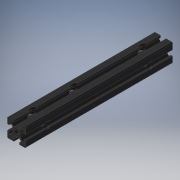
# Autodesk Inventor part: HFS5-2020-160-AH24-BH136-Z6-XA20-XB65-XC140
Saved by Autodesk Inventor 2019 (Build 230136000, 136)
## iProperties
Created: 2024-09-09
Part Number: HFS5-2020-160-AH24-BH136-Z6-XA20-XB65-XC140
Material: Generic
Catalog Web Link: www.cadenas.de
Description: NFS5-2020, NFSB5-2020, HFS5-2020, HFSB5-2020, CAF5-2020, HFSY5-2020, NFSF5-2020, HFSF5-2020, HFSFB5-2020, NFST5-2020, HFST5-2020, HFSTB5-2020, HFSH5-2020, HFSC5-2020-HFS5 Series Aluminum Extrusions 20 Square -1 Slot-
Vendor: MISUMI
Document SubType Name: Modeling
Designer: psAdmin
Manufacturer: MISUMI
Mass: 27.8589 g
Surface Area: 278.381 cm^2
Volume: 27.8589 cm^3
Density: 1 g/cm^3
Appearance: PSOLRGB-175-175-175
Category: PARTsolutions
Company: MISUMI
Title: HFS5-2020-160-AH24-BH136-Z6-XA20-XB65-XC140
Author: Cadenas PARTsolutions
Comments: HFS5 Series Aluminum Extrusions 20 Square -1 Slot-
PSOL_IDENT_0: {$CADENAS_DATA/23d-libs/misumi/metric/38_al_extrusions_blackets/5/hfs5_2020.prj},737 {VTYP=3D},{NB=H
PSOL_IDENT_1: FS5-2020-160-AH24-BH136-Z6-XA20-XB65-XC140},{LINA=HFS5-2020-160-AH24-BH136-Z6-XA20-XB65-XC140},{NN=N
PSOL_IDENT_2: FS5-2020, NFSB5-2020, HFS5-2020, HFSB5-2020, CAF5-2020, HFSY5-2020, NFSF5-2020, HFSF5-2020, HFSFB5-2
PSOL_IDENT_3: 020, NFST5-2020, HFST5-2020, HFSTB5-2020, HFSH5-2020, HFSC5-2020},{DATE=08.05.2023 08:39:06},{GEOMDA
PSOL_IDENT_4: TE=27.07.2021 03:20:00},{VERSION=},{LINEID=150},{WBVAR=L,ALT1,ALT2,ALT4,ALT5,CP5,DL5,DR5,ALT6,ALT9,A
PSOL_IDENT_5: LT10,ALT11,HP6,NHL6,DL6,NHR6,DR6,ALT7,ALT8,NH9,AH,BH,CH,DH,EH,NH10,AV,BV,CV,DV,EV,NH11,AP,BP,CP,DP,E
PSOL_IDENT_6: P,ALT12,ALT13,Z,NH12,XA,XB,XC,XD,XE,NH13,YA,YB,YC,YD,YE,ALT16,HP16,DL16,DR16,ALT17,HQ17,JLP,ALT20},{
PSOL_IDENT_7: WBNUMERIC=L,NH9,AH,BH,CH,DH,EH,NH10,AV,BV,CV,DV,EV,NH11,AP,BP,CP,DP,EP,NH12,XA,XB,XC,XD,XE,NH13,YA,Y
PSOL_IDENT_8: B,YC,YD,YE,HQ17,JLP}  {NB=HFS5-2020-160-AH24-BH136-Z6-XA20-XB65-XC140},{LINA=HFS5-2020-160-AH24-BH13
PSOL_IDENT_9: 6-Z6-XA20-XB65-XC140},{KT=DUMMY},{PN=HFS5-2020-160-AH24-BH136-Z6-XA20-XB65-XC140},{TPS=HFS5-2020},{M
PSOL_IDENT_10: AT=A6N01SS-T5 Aluminum Alloy or 6005A-T5 Aluminum Alloy},{ST=Clear Anodize},{FRMW=20},{FRMH=20},{FRD=
PSOL_IDENT_11: 4.2},{L=160},{MASS=0.5},{SA=183},{LX=0.742x10^4},{LY=0.742x10^4},{ALT1=},{M1=0},{DPL1=0},{DPR1=0},{A
PSOL_IDENT_12: LT1PN=},{ALT2=},{ALT2ALG= '','w/o End Tapping (Heli-Coil Insert)','LHP','with LHP (Tapping on the Le
PSOL_IDENT_13: ft (Heli-Coil Insert))','RHP','with RHP (Tapping on the Right (Heli-Coil Insert))','HPW','with HPW (
PSOL_IDENT_14: Tapping on Both Ends (Heli-Coil Insert))' },{M2=0},{DP2=0},{ALT2PN=},{ALT4=},{ALT4ALG= '', 'w/o SC (
PSOL_IDENT_15: High Precision Cut)', 'SC', 'with SC (High Precision Cut)' },{ALT4PN=},{ALT5=},{ALT5ALG= '','w/o 45
PSOL_IDENT_16: Degree Cut','1','with 45 Degree Cut' },{CP5=},{CP5ALG= '','N/A' },{DL5=},{DL5ALG= '','N/A' },{DR5=},
PSOL_IDENT_17: {DR5ALG= '','N/A' },{FRMLALT5=0},{FRMRALT5=0},{ALT5PN=},{ALT6=},{ALT6ALG= '','w/o Fastening Location
PSOL_IDENT_18: Wrench Access Hole Alterations','1','with Fastening Location Wrench Access Hole Alterations' },{ALT
PSOL_IDENT_19: 9=1},{ALT9ALG= '','w/o Location Specified Wrench Access Hole Alteratons (Horizontal)','1','with Loca
PSOL_IDENT_20: tion Specified Wrench Access Hole Alteratons (Horizontal)' },{ALT10=},{ALT10ALG= '','w/o Location Sp
PSOL_IDENT_21: ecified Wrench Access Hole Alteratons (Vertical)','1','with Location Specified Wrench Access Hole Al
PSOL_IDENT_22: teratons (Vertical)' },{ALT11=},{ALT11ALG= '','w/o Location Specified Wrench Access Hole Alteratons
PSOL_IDENT_23: (Crisscross)','1','with Location Specified Wrench Access Hole Alteratons (Crisscross)' },{HP6=},{HP6
PSOL_IDENT_24: ALG= '','N/A' },{NHL6=},{NHL6ALG= '','N/A' },{DL6=},{DL6ALG= '','N/A' },{NHR6=},{NHR6ALG= '','N/A' }
PSOL_IDENT_25: ,{DR6=},{DR6ALG= '','N/A' },{HL6=0.000},{HL6D=0},{HR6=0.000},{HR6D=0},{J6=0},{J6D=0},{K6=0},{K6D=0},
PSOL_IDENT_26: {DD6=7.35},{DD6ALG=7.35},{ALT7=},{ALT7ALG= '','N/A' },{ALT8=},{ALT8ALG= '','N/A' },{ALT678PN=},{NH9=
PSOL_IDENT_27: 2},{NH9MAX=5},{NH9ALG=[1:5/1]},{AH=24.0},{AHMIN=7},{AHMAX=143.5},{AHALG=[7:143.5/0.5]},{BH=136.0},{B
PSOL_IDENT_28: HMIN=33.5},{BHMAX=153},{BHALG=[33.5:153/0.5]},{CH=0.0},{CHMIN=145.5},{CHMAX=162.5},{CHALG=[0]},{DH=0
PSOL_IDENT_29: .0},{DHMIN=9.5},{DHMAX=172},{DHALG=[0]},{EH=0.0},{EHMIN=9.5},{EHMAX=153},{EHALG=[0]},{NH10=0},{NH10M
PSOL_IDENT_30: AX=5},{NH10ALG=[0]},{AV=0.0},{AVMIN=7},{AVMAX=162.5},{AVALG=[0]},{BV=0.0},{BVMIN=9.5},{BVMAX=172},{B
PSOL_IDENT_31: VALG=[0]},{CV=0.0},{CVMIN=9.5},{CVMAX=181.5},{CVALG=[0]},{DV=0.0},{DVMIN=9.5},{DVMAX=191},{DVALG=[0]
PSOL_IDENT_32: },{EV=0.0},{EVMIN=9.5},{EVMAX=153},{EVALG=[0]},{NH11=0},{NH11MAX=5},{NH11ALG=[0]},{AP=0.0},{APMIN=7}
PSOL_IDENT_33: ,{APMAX=162.5},{APALG=[0]},{BP=0.0},{BPMIN=9.5},{BPMAX=172},{BPALG=[0]},{CP=0.0},{CPMIN=9.5},{CPMAX=
PSOL_IDENT_34: 181.5},{CPALG=[0]},{DP=0.0},{DPMIN=9.5},{DPMAX=191},{DPALG=[0]},{EP=0.0},{EPMIN=9.5},{EPMAX=153},{EP
PSOL_IDENT_35: ALG=[0]},{ALT9PN=-AH24-BH136},{ALT10PN=},{ALT11PN=},{ALT91011PN=-AH24-BH136},{ALT12=1},{ALT12ALG= ''
PSOL_IDENT_36: ,'w/o Counterbore Hole in Specified Position (Vertical)','1','with Counterbore Hole in Specified Pos
PSOL_IDENT_37: ition (Vertical)' },{ALT13=},{ALT13ALG= '','w/o Counterbore Hole in Specified Position (Horizontal)'
PSOL_IDENT_38: ,'1','with Counterbore Hole in Specified Position (Horizontal)' },{Z=6},{ZALG='5','5','6','6'},{DD12=
PSOL_IDENT_39: 6.5},{DD112=11.0},{NH12=3},{NH12MAX=5},{NH12ALG=[1:5/1]},{XA=20.0},{XAMIN=7},{XAMAX=127},{XAALG=[7:1
PSOL_IDENT_40: 27/0.5]},{XB=65.0},{XBMIN=33},{XBMAX=140},{XBALG=[33:140/0.5]},{XC=140.0},{XCMIN=78},{XCMAX=153},{XC
PSOL_IDENT_41: ALG=[78:153/0.5]},{XD=0.0},{XDMIN=153},{XDMAX=166},{XDALG=[0]},{XE=0.0},{XEMIN=13},{XEMAX=153},{XEAL
PSOL_IDENT_42: G=[0]},{NH13=0},{NH13MAX=5},{NH13ALG=[0]},{YA=0.0},{YAMIN=7},{YAMAX=166},{YAALG=[0]},{YB=0.0},{YBMIN=
PSOL_IDENT_43: 13},{YBMAX=179},{YBALG=[0]},{YC=0.0},{YCMIN=13},{YCMAX=192},{YCALG=[0]},{YD=0.0},{YDMIN=13},{YDMAX=2
PSOL_IDENT_44: 05},{YDALG=[0]},{YE=0.0},{YEMIN=13},{YEMAX=153},{YEALG=[0]},{ALT12PN=-XA20-XB65-XC140},{ALT13PN=},{A
PSOL_IDENT_45: LT1213PN=-Z6-XA20-XB65-XC140},{ALT16=},{ALT16ALG= '','w/o M Type Hole Alteration','1','with M Type H
PSOL_IDENT_46: ole Alteration' },{HP16=},{HP16ALG= '','N/A' },{DL16=},{DL16ALG= '','N/A' },{DR16=},{DR16ALG= '','N/
PSOL_IDENT_47: A' },{H116=0},{D16=0.0},{ALT16PN=},{ALT17=},{ALT17ALG= '','w/o L Type Hole Alteration (Top)','1','wi
PSOL_IDENT_48: th L Type Hole Alteration (Top)' },{HQ17=0},{HQ17ALG=0},{JLP=0},{JLPMIN=4.9},{JLPMAX=0},{JLPALG=[0]}
PSOL_IDENT_49: ,{L17=0},{D17=0.0},{ALT17PN=},{ALT20=},{ALT20PN=},{ERRORALT01=OK},{ERRORALT02=OK},{ERRORALT05=OK},{E
PSOL_IDENT_50: RRORALT06091=OK},{ERRORALT06092=OK},{ERRORALT06093=OK},{ERRORALT06094=OK},{ERRORALT06101=OK},{ERRORA
PSOL_IDENT_51: LT06102=OK},{ERRORALT06103=OK},{ERRORALT06104=OK},{ERRORALT06111=OK},{ERRORALT06112=OK},{ERRORALT061
PSOL_IDENT_52: 13=OK},{ERRORALT06114=OK},{ERRORALT06121=OK},{ERRORALT06122=OK},{ERRORALT06123=OK},{ERRORALT06124=OK
PSOL_IDENT_53: },{ERRORALT06131=OK},{ERRORALT06132=OK},{ERRORALT06133=OK},{ERRORALT06134=OK},{ERRORALT0616=OK},{ERR
PSOL_IDENT_54: ORALT06171=OK},{ERRORALT06172=OK},{ERRORALT06173=OK},{ERRORALT0911=OK},{ERRORALT0913=OK},{ERRORALT09
PSOL_IDENT_55: 16=OK},{ERRORALT0917=OK},{ERRORALT1011=OK},{ERRORALT1012=OK},{ERRORALT1016=OK},{ERRORALT1017=OK},{ER
PSOL_IDENT_56: RORALT1112=OK},{ERRORALT1113=OK},{ERRORALT1116=OK},{ERRORALT1117=OK},{ERRORALT1216=OK},{ERRORALT1217=
PSOL_IDENT_57: OK},{ERRORALT1316=OK},{ERRORALT1317=OK},{ERRORALT1617=OK},{ERRORPN=},{TFW=0}
NB: HFS5-2020-160-AH24-BH136-Z6-XA20-XB65-XC140
NN: NFS5-2020, NFSB5-2020, HFS5-2020, HFSB5-2020, CAF5-2020, HFSY5-2020, NFSF5-2020, HFSF5-2020, HFSFB5-2020, NFST5-2020, HFST5-2020, HFSTB5-2020, HFSH5-2020, HFSC5-2020
NT: HFS5 Series Aluminum Extrusions 20 Square -1 Slot-
NBSYN: $PN.
LINA: HFS5-2020-160-AH24-BH136-Z6-XA20-XB65-XC140
CATALOG: Misumi
PN: HFS5-2020-160-AH24-BH136-Z6-XA20-XB65-XC140
TPS: HFS5-2020
MAT: A6N01SS-T5 Aluminum Alloy or 6005A-T5 Aluminum Alloy
ST: Clear Anodize
L: 160
MASS: 0.5
SA: 183
LX: 0.742x10^4
LY: 0.742x10^4
ALT1: w/o End Tapping
M1: 0
DPL1: 0
DPR1: 0
ALT2: w/o End Tapping (Heli-Coil Insert)
M2: 0
DP2: 0
ALT4: w/o SC (High Precision Cut)
ALT5: w/o 45 Degree Cut
CP5: N/A
DL5: N/A
DR5: N/A
ALT6: w/o Fastening Location Wrench Access Hole Alterations
ALT9: with Location Specified Wrench Access Hole Alteratons (Horizontal)
ALT10: w/o Location Specified Wrench Access Hole Alteratons (Vertical)
ALT11: w/o Location Specified Wrench Access Hole Alteratons (Crisscross)
HP6: N/A
NHL6: N/A
DL6: N/A
NHR6: N/A
DR6: N/A
HL6D: 0
HR6D: 0
J6D: 0
K6D: 0
DD6: 7.35
ALT7: N/A
ALT8: N/A
NH9: 2
AH: 24
BH: 136
CH: 0
DH: 0
EH: 0
NH10: 0
AV: 0
BV: 0
CV: 0
DV: 0
EV: 0
NH11: 0
AP: 0
BP: 0
CP: 0
DP: 0
EP: 0
ALT12: with Counterbore Hole in Specified Position (Vertical)
ALT13: w/o Counterbore Hole in Specified Position (Horizontal)
Z: 6
DD12: 6.5
DD112: 11
NH12: 3
XA: 20
XB: 65
XC: 140
XD: 0
XE: 0
NH13: 0
YA: 0
YB: 0
YC: 0
YD: 0
YE: 0
ALT16: w/o M Type Hole Alteration
HP16: N/A
DL16: N/A
DR16: N/A
H116: 0
D16: 0
ALT17: w/o L Type Hole Alteration (Top)
HQ17: 0
JLP: 0
D17: 0
ALT20: w/o CW (End Face C Chamfering)
SUPPLIER: MISUMI
ARTICLENO: HFS5-2020-160-AH24-BH136-Z6-XA20-XB65-XC140
BOMINFO: HFS5-2020-160-AH24-BH136-Z6-XA20-XB65-XC140
CREATOR: CADENAS GmbH
Autodesk Inventor part; units mm, degrees
sketch "Sketch_1" plane through (0, 0, 0) normal (0, 0, 1) x (1, 0, 0)
  line L0 (-10, -3) -> (-10, -9)
  arc A0 (-10, -9) -> (-9, -10) centre (-9, -9) ccw
  line L1 (-9, -10) -> (-3, -10)
  line L2 (-3, -10) -> (-3, -8)
  line L3 (-3, -8) -> (-6, -8)
  line L4 (-6, -8) -> (-6, -7.0607)
  line L5 (-6, -7.0607) -> (-2.9393, -4)
  line L6 (-2.9393, -4) -> (-0.5196, -4)
  line L7 (-0.5196, -4) -> (0, -3.7)
  line L8 (0, -3.7) -> (0.5196, -4)
  line L9 (0.5196, -4) -> (2.9393, -4)
  line L10 (2.9393, -4) -> (6, -7.0607)
  line L11 (6, -7.0607) -> (6, -8)
  line L12 (6, -8) -> (3, -8)
  line L13 (3, -8) -> (3, -10)
  line L14 (3, -10) -> (9, -10)
  arc A1 (9, -10) -> (10, -9) centre (9, -9) ccw
  line L15 (10, -9) -> (10, -3)
  line L16 (10, -3) -> (8, -3)
  line L17 (8, -3) -> (8, -6)
  line L18 (8, -6) -> (7.0607, -6)
  line L19 (7.0607, -6) -> (4, -2.9393)
  line L20 (4, -2.9393) -> (4, -0.5196)
  line L21 (4, -0.5196) -> (3.7, 0)
  line L22 (3.7, 0) -> (4, 0.5196)
  line L23 (4, 0.5196) -> (4, 2.9393)
  line L24 (4, 2.9393) -> (7.0607, 6)
  line L25 (7.0607, 6) -> (8, 6)
  line L26 (8, 6) -> (8, 3)
  line L27 (8, 3) -> (10, 3)
  line L28 (10, 3) -> (10, 9)
  arc A2 (10, 9) -> (9, 10) centre (9, 9) ccw
  line L29 (9, 10) -> (3, 10)
  line L30 (3, 10) -> (3, 8)
  line L31 (3, 8) -> (6, 8)
  line L32 (6, 8) -> (6, 7.0607)
  line L33 (6, 7.0607) -> (2.9393, 4)
  line L34 (2.9393, 4) -> (0.5196, 4)
  line L35 (0.5196, 4) -> (0, 3.7)
  line L36 (0, 3.7) -> (-0.5196, 4)
  line L37 (-0.5196, 4) -> (-2.9393, 4)
  line L38 (-2.9393, 4) -> (-6, 7.0607)
  line L39 (-6, 7.0607) -> (-6, 8)
  line L40 (-6, 8) -> (-3, 8)
  line L41 (-3, 8) -> (-3, 10)
  line L42 (-3, 10) -> (-9, 10)
  arc A3 (-9, 10) -> (-10, 9) centre (-9, 9) ccw
  line L43 (-10, 9) -> (-10, 3)
  line L44 (-10, 3) -> (-8, 3)
  line L45 (-8, 3) -> (-8, 6)
  line L46 (-8, 6) -> (-7.0607, 6)
  line L47 (-7.0607, 6) -> (-4, 2.9393)
  line L48 (-4, 2.9393) -> (-4, 0.5196)
  line L49 (-4, 0.5196) -> (-3.7, 0)
  line L50 (-3.7, 0) -> (-4, -0.5196)
  line L51 (-4, -0.5196) -> (-4, -2.9393)
  line L52 (-4, -2.9393) -> (-7.0607, -6)
  line L53 (-7.0607, -6) -> (-8, -6)
  line L54 (-8, -6) -> (-8, -3)
  line L55 (-8, -3) -> (-10, -3)
  constraints: 112 end point, 8 point on circle, 4 centre point
extrude "Extrusion1" add sketch "Sketch_1" against normal blind 160
sketch "Sketch2" plane through (0, 0, -160) normal (0, 0, -1) x (-1, 0, 0)
  point P0 (0, 0)
hole "Hole1" at (0, 0, -160) direction (0, 0, 1) diameter 4.2 depth 160
sketch "Sketch_62" plane through (0, 0, 0) normal (0, 1, 0) x (1, 0, 0)
  line L0 (10, 24) -> (-10, 24)
  line L1 (-10, 24) -> (-10, 27.675)
  line L2 (-10, 27.675) -> (10, 27.675)
  line L3 (10, 27.675) -> (10, 24)
  line L4 (10, 24) -> (-10, 24)
  constraints: 10 end point
revolve "Revolution1" cut sketch "Sketch_62" angle 360 about axis through (10, 0, -24) along (1, 0, 0)
sketch "Sketch_25" plane through (0, 0, 0) normal (0, 1, 0) x (1, 0, 0)
  line L0 (10, 136) -> (-10, 136)
  line L1 (-10, 136) -> (-10, 139.675)
  line L2 (-10, 139.675) -> (10, 139.675)
  line L3 (10, 139.675) -> (10, 136)
  line L4 (10, 136) -> (-10, 136)
  constraints: 10 end point
revolve "Revolution2" cut sketch "Sketch_25" angle 360 about axis through (10, 0, -136) along (1, 0, 0)
sketch "Sketch_30" plane through (0, 0, 0) normal (1, 0, 0) x (0, 0, -1)
  line L0 (20, -10) -> (20, 10)
  line L1 (20, 10) -> (25.5, 10)
  line L2 (25.5, 10) -> (25.5, 4)
  line L3 (25.5, 4) -> (23.25, 4)
  line L4 (23.25, 4) -> (23.25, -10)
  line L5 (23.25, -10) -> (20, -10)
  line L6 (20, -10) -> (20, 10)
  constraints: 14 end point
revolve "Revolution3" cut sketch "Sketch_30" angle 360 about axis through (0, -10, -20) along (0, -1, 0)
sketch "Sketch_31" plane through (0, 0, 0) normal (1, 0, 0) x (0, 0, -1)
  line L0 (65, -10) -> (65, 10)
  line L1 (65, 10) -> (70.5, 10)
  line L2 (70.5, 10) -> (70.5, 4)
  line L3 (70.5, 4) -> (68.25, 4)
  line L4 (68.25, 4) -> (68.25, -10)
  line L5 (68.25, -10) -> (65, -10)
  line L6 (65, -10) -> (65, 10)
  constraints: 14 end point
revolve "Revolution4" cut sketch "Sketch_31" angle 360 about axis through (0, -10, -65) along (0, -1, 0)
sketch "Sketch_47" plane through (0, 0, 0) normal (1, 0, 0) x (0, 0, -1)
  line L0 (140, -10) -> (140, 10)
  line L1 (140, 10) -> (145.5, 10)
  line L2 (145.5, 10) -> (145.5, 4)
  line L3 (145.5, 4) -> (143.25, 4)
  line L4 (143.25, 4) -> (143.25, -10)
  line L5 (143.25, -10) -> (140, -10)
  line L6 (140, -10) -> (140, 10)
  constraints: 14 end point
revolve "Revolution5" cut sketch "Sketch_47" angle 360 about axis through (0, -10, -140) along (0, -1, 0)
ref_plane "C1_XY" through (0, 0, 0) normal (0, 0, 1) x (1, 0, 0)
ref_plane "C1_YZ" through (0, 0, 0) normal (1, 0, 0) x (0, 1, 0)
ref_plane "C1_ZX" through (0, 0, 0) normal (0, 1, 0) x (0, 0, 1)
body "Solid1"
